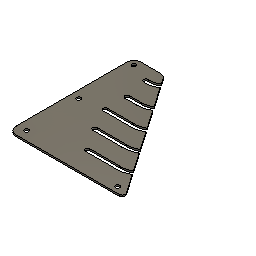
Rullateline v4 (Autodesk Fusion 360 design; units mm, degrees)
Autodesk Fusion 360 part; units mm, degrees
sketch "Sketch1" plane through (0, 0, 0) normal (0, 1, 0) x (1, 0, 0)
  line L0 (0, 0) -> (0, 830)
  line L1 (0, 830) -> (200, 830)
  line L2 (0, 0) -> (770, 0)
  line L3 (770, 0) -> (200, 830)
  dimension "d1" = 830
  dimension "d2" = 770
  measures "d1" distance of L0.start
  measures "d2" distance of L0.start
extrude "Extrude1" add sketch "Sketch1" along normal blind 11
sketch "Sketch2" plane through (0, 11, 0) normal (0, 1, 0) x (-1, 0, 0)
  line L0 (0, 0) -> (-770, 0)
  line L1 (-770, 0) -> (-200, -830)
  line L2 (-200, -830) -> (0, -830)
  line L3 (0, -830) -> (0, 0)
  arc A0 (-167.9783, -725.6164) -> (-256.5823, -748.2599) centre (-183.687, -848.8237) ccw
  arc A1 (-171.646, -754.3836) -> (-167.9783, -725.6164) centre (-169.8121, -740) ccw
  arc A2 (-171.646, -754.3836) -> (-239.5623, -771.7401) centre (-183.687, -848.8237) ccw
  arc A3 (-256.5823, -748.2599) -> (-239.5623, -771.7401) centre (-248.0723, -760) ccw
  arc A4 (-169.8121, -740) -> (-248.0723, -760) centre (-183.687, -848.8237) ccw construction
  arc A5 (-277.8741, -599.4877) -> (-346.9644, -617.3771) centre (-282.9401, -722.2833) ccw
  arc A6 (-277.8741, -599.4877) -> (-276.6787, -570.5123) centre (-277.2764, -585) ccw
  arc A7 (-276.6787, -570.5123) -> (-362.0718, -592.6229) centre (-282.9401, -722.2833) ccw
  arc A8 (-362.0718, -592.6229) -> (-346.9644, -617.3771) centre (-354.5181, -605) ccw
  arc A9 (-277.2764, -585) -> (-354.5181, -605) centre (-282.9401, -722.2833) ccw construction
  arc A10 (-370.6712, -454.4432) -> (-446.4891, -472.3442) centre (-381.6102, -577.6218) ccw
  arc A11 (-370.6712, -454.4432) -> (-368.1059, -425.5568) centre (-369.3886, -440) ccw
  arc A12 (-368.1059, -425.5568) -> (-461.7037, -447.6558) centre (-381.6102, -577.6218) ccw
  arc A13 (-461.7037, -447.6558) -> (-446.4891, -472.3442) centre (-454.0964, -460) ccw
  arc A14 (-369.3886, -440) -> (-454.0964, -460) centre (-381.6102, -577.6218) ccw construction
  arc A15 (-470.9702, -309.4832) -> (-546.4851, -327.592) centre (-477.6426, -448.1642) ccw
  arc A16 (-470.9702, -309.4832) -> (-469.5765, -280.5168) centre (-470.2734, -295) ccw
  arc A17 (-469.5765, -280.5168) -> (-560.8643, -302.408) centre (-477.6426, -448.1642) ccw
  arc A18 (-560.8643, -302.408) -> (-546.4851, -327.592) centre (-553.6747, -315) ccw
  arc A19 (-470.2734, -295) -> (-553.6747, -315) centre (-477.6426, -448.1642) ccw construction
  arc A20 (-574.3852, -164.4572) -> (-645.4659, -182.2316) centre (-583.2764, -279.9159) ccw
  arc A21 (-574.3852, -164.4572) -> (-572.1585, -135.5428) centre (-573.2718, -150) ccw
  arc A22 (-572.1585, -135.5428) -> (-661.0401, -157.7684) centre (-583.2764, -279.9159) ccw
  arc A23 (-661.0401, -157.7684) -> (-645.4659, -182.2316) centre (-653.253, -170) ccw
  arc A24 (-573.2718, -150) -> (-653.253, -170) centre (-583.2764, -279.9159) ccw construction
  line L4 (-573.2718, -164.5) -> (-373.7749, -164.5)
  arc A25 (-373.7749, -164.5) -> (-373.7749, -135.5) centre (-373.7749, -150) ccw
  line L5 (-373.7749, -135.5) -> (-573.2718, -135.5)
  arc A26 (-573.2718, -135.5) -> (-573.2718, -164.5) centre (-573.2718, -150) ccw
  line L6 (-573.2718, -150) -> (-373.7749, -150) construction
  line L7 (-470.2734, -309.5) -> (-277.2764, -309.5)
  arc A27 (-277.2764, -309.5) -> (-277.2764, -280.5) centre (-277.2764, -295) ccw
  line L8 (-277.2764, -280.5) -> (-470.2734, -280.5)
  arc A28 (-470.2734, -280.5) -> (-470.2734, -309.5) centre (-470.2734, -295) ccw
  line L9 (-470.2734, -295) -> (-277.2764, -295) construction
  line L10 (-369.3886, -454.5) -> (-200, -454.5)
  arc A29 (-200, -454.5) -> (-200, -425.5) centre (-200, -440) ccw
  line L11 (-200, -425.5) -> (-369.3886, -425.5)
  arc A30 (-369.3886, -425.5) -> (-369.3886, -454.5) centre (-369.3886, -440) ccw
  line L12 (-369.3886, -440) -> (-200, -440) construction
  line L13 (-277.2764, -599.5) -> (-200, -599.5)
  arc A31 (-200, -599.5) -> (-200, -570.5) centre (-200, -585) ccw
  line L14 (-200, -570.5) -> (-277.2764, -570.5)
  arc A32 (-277.2764, -570.5) -> (-277.2764, -599.5) centre (-277.2764, -585) ccw
  line L15 (-277.2764, -585) -> (-200, -585) construction
  dimension "d13" = 90
  dimension "d14" = 245
  dimension "d15" = 390
  dimension "d16" = 390
  dimension "d17" = 535
  dimension "d18" = 535
  dimension "d19" = 680
  dimension "d20" = 680
  dimension "d21" = 29
  dimension "d22" = 29
  dimension "d23" = 29
  dimension "d24" = 29
  dimension "d25" = 29
  dimension "d26" = 20
  dimension "d27" = 20
  dimension "d28" = 20
  dimension "d29" = 20
  dimension "d30" = 20
  dimension "d31" = 29
  dimension "d32" = 29
  dimension "d33" = 29
  dimension "d40" = 29
  measures "d13" distance of L2
  measures "d14" distance of L2
  measures "d15" distance of L2
  measures "d16" distance of L2
  measures "d17" distance of L2
  measures "d18" distance of L2 L0.start
  measures "d19" distance of L2
  measures "d20" distance of L2
  measures "d21" diameter of A3
  measures "d22" diameter of A6
  measures "d23" diameter of A11
  measures "d24" diameter of A16
  measures "d25" diameter of A21
  measures "d31" diameter of A25
  measures "d32" diameter of A27
  measures "d33" diameter of A29
  measures "d40" diameter of A31
extrude "Extrude2" cut sketch "Sketch2" against normal blind 12 contours L1 A20 A22 A23 L5 A26 | L1 A20 A23 | L1 A0 A3 | L1 A0 A1 A2 A3 | L1 A15 A17 A18 L8 A28 | L1 A15 A18 | A21 A22 L5 A26 | A21 A22 L4 A25 L5 | L1 A5 A8 | L1 A5 A7 A8 L14 A32 | L1 A10 A12 A13 L11 A30 | L1 A10 A13 | A16 A17 L8 A28 | A16 A17 L7 A27 L8 | A6 A7 L14 A32 | A11 A12 L11 A30 | A11 A12 L10 A29 L11
fillet "Fillet1" radius 50 1 edges at (0, 5.5, -830)
fillet "Fillet2" radius 50 1 edges at (200, 5.5, -830)
fillet "Fillet3" radius 50 1 edges at (0, 5.5, 0)
fillet "Fillet4" radius 20 1 edges at (770, 5.5, 0)
extrude "Extrude3" cut sketch "Sketch2" against normal blind 12 contours A6 A7 L13 A31 L14
sketch "Sketch3" plane through (0, 11, 0) normal (0, 1, 0) x (-1, 0, 0)
  line L0 (-276.9849, -570.5) -> (-200, -570.5)
  arc A0 (-200, -599.5) -> (-200, -570.5) centre (-200, -585) ccw
  line L1 (-200, -599.5) -> (-277.2764, -599.5)
  arc A1 (-277.8741, -599.4877) -> (-277.2764, -599.5) centre (-277.2764, -585) ccw
  arc A2 (-277.8741, -599.4877) -> (-346.2962, -616.9722) centre (-282.9401, -722.2833) ccw
  line L2 (-346.2962, -616.9722) -> (-256.2832, -748.0438)
  arc A3 (-167.9783, -725.6164) -> (-256.2832, -748.0438) centre (-183.687, -848.8237) ccw
  arc A4 (-171.646, -754.3836) -> (-167.9783, -725.6164) centre (-169.8121, -740) ccw
  arc A5 (-171.646, -754.3836) -> (-239.5623, -771.7401) centre (-183.687, -848.8237) ccw
  arc A6 (-239.8637, -771.9528) -> (-239.5623, -771.7401) centre (-248.0723, -760) ccw
  line L3 (-239.8637, -771.9528) -> (-214.8987, -808.3054)
  arc A7 (-214.8987, -808.3054) -> (-173.6821, -830) centre (-173.6821, -780) ccw
  line L4 (-173.6821, -830) -> (-50, -830)
  arc A8 (-50, -830) -> (0, -780) centre (-50, -780) ccw
  line L5 (0, -780) -> (0, -50)
  arc A9 (0, -50) -> (-50, 0) centre (-50, -50) ccw
  line L6 (-50, 0) -> (-732.003, 0)
  arc A10 (-732.003, 0) -> (-748.4896, -31.3221) centre (-732.003, -20) ccw
  line L7 (-748.4896, -31.3221) -> (-661.4616, -158.0472)
  arc A11 (-661.0401, -157.7684) -> (-661.4616, -158.0472) centre (-653.253, -170) ccw
  arc A12 (-572.7291, -135.5) -> (-661.0401, -157.7684) centre (-583.2764, -279.9159) ccw
  line L8 (-572.7291, -135.5) -> (-373.7749, -135.5)
  arc A13 (-373.7749, -164.5) -> (-373.7749, -135.5) centre (-373.7749, -150) ccw
  line L9 (-373.7749, -164.5) -> (-573.2718, -164.5)
  arc A14 (-574.3852, -164.4572) -> (-573.2718, -164.5) centre (-573.2718, -150) ccw
  arc A15 (-574.3852, -164.4572) -> (-645.0388, -181.961) centre (-583.2764, -279.9159) ccw
  line L10 (-645.0388, -181.961) -> (-561.8833, -303.0472)
  arc A16 (-560.8643, -302.408) -> (-561.8833, -303.0472) centre (-553.6747, -315) ccw
  arc A17 (-469.9326, -280.5) -> (-560.8643, -302.408) centre (-477.6426, -448.1642) ccw
  line L11 (-469.9326, -280.5) -> (-277.2764, -280.5)
  arc A18 (-277.2764, -309.5) -> (-277.2764, -280.5) centre (-277.2764, -295) ccw
  line L12 (-277.2764, -309.5) -> (-470.2734, -309.5)
  arc A19 (-470.9702, -309.4832) -> (-470.2734, -309.5) centre (-470.2734, -295) ccw
  arc A20 (-470.9702, -309.4832) -> (-545.4348, -326.9984) centre (-477.6426, -448.1642) ccw
  line L13 (-545.4348, -326.9984) -> (-462.3049, -448.0472)
  arc A21 (-461.7037, -447.6558) -> (-462.3049, -448.0472) centre (-454.0964, -460) ccw
  arc A22 (-368.762, -425.5) -> (-461.7037, -447.6558) centre (-381.6102, -577.6218) ccw
  line L14 (-368.762, -425.5) -> (-200, -425.5)
  arc A23 (-200, -454.5) -> (-200, -425.5) centre (-200, -440) ccw
  line L15 (-200, -454.5) -> (-369.3886, -454.5)
  arc A24 (-370.6712, -454.4432) -> (-369.3886, -454.5) centre (-369.3886, -440) ccw
  arc A25 (-370.6712, -454.4432) -> (-445.8766, -471.9692) centre (-381.6102, -577.6218) ccw
  line L16 (-445.8766, -471.9692) -> (-362.7266, -593.0472)
  arc A26 (-362.0718, -592.6229) -> (-362.7266, -593.0472) centre (-354.5181, -605) ccw
  arc A27 (-276.9849, -570.5) -> (-362.0718, -592.6229) centre (-282.9401, -722.2833) ccw
  circle A28 centre (-40, -790) radius 13.9
  circle A29 centre (-60, -60) radius 13.9
  circle A30 centre (-682.712, -40) radius 13.9
  circle A31 centre (-50, -415) radius 13.9
  dimension "d43" = 27.8
  dimension "d44" = 40
  dimension "d45" = 40
  dimension "d46" = 27.8
  dimension "d47" = 27.8
  dimension "d48" = 60
  dimension "d49" = 60
  dimension "d50" = 40
  dimension "d51" = 27.8
  dimension "d52" = 50
  dimension "d53" = 415
  measures "d43" diameter of A28
  measures "d44" distance of L4
  measures "d45" distance of L5
  measures "d46" diameter of A29
  measures "d47" diameter of A30
  measures "d48" distance of L6 origin
  measures "d49" distance of L5 origin
  measures "d50" distance of L6
  measures "d51" diameter of A31
  measures "d52" distance of L5
  measures "d53" distance of L6
extrude "Extrude4" cut sketch "Sketch3" against normal blind 12 contours A28 | A29 | A30 | A31
